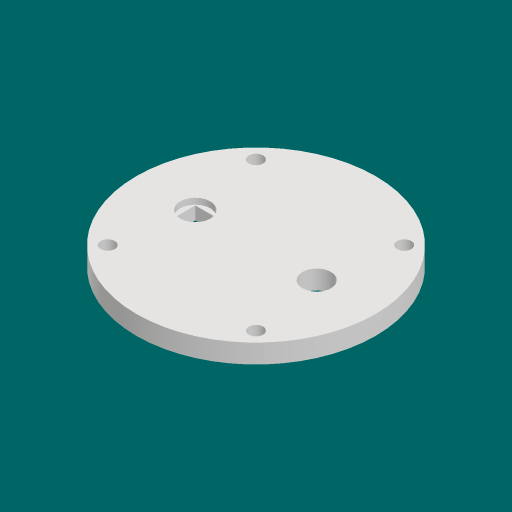
# Autodesk Inventor part: carriage
Saved by Autodesk Inventor 2023.1 (Build 271208000, 208)
## iProperties
Created: 2022-10-10
Part Number: carriage
Material: Generic
Document SubType Name: Modeling
Designer: zac-h
Density: 1 g/cm^3
Appearance: Default
Author: zac-h
Autodesk Inventor part; units mm, degrees
ref_plane "YZ Plane" through (0, 0, 0) normal (1, 0, 0) x (0, 1, 0)
ref_plane "XZ Plane" through (0, 0, 0) normal (0, 1, 0) x (-1, 0, 0)
ref_plane "XY Plane" through (0, 0, 0) normal (0, 0, 1) x (1, 0, 0)
sketch "Sketch1" plane through (0, 0, 0) normal (0, 1, 0) x (-1, 0, 0)
  point P0 (0, 0)
sketch "Sketch2" plane through (0, 0, 0) normal (0, 1, 0) x (-1, 0, 0)
  circle A0 centre (0, 0) radius 4.7625
  circle A1 centre (20.32, 0) radius 40
  line L0 (20.32, -34.925) -> (20.32, 34.925) construction
  line L1 (29.845, -25.4) -> (29.845, 25.4) construction
  line L2 (10.795, 25.4) -> (10.795, -25.4) construction
  arc A2 (10.795, -25.4) -> (29.845, -25.4) centre (20.32, -25.4) ccw construction
  arc A3 (29.845, 25.4) -> (10.795, 25.4) centre (20.32, 25.4) ccw construction
  line L3 (-19.68, 0) -> (60.32, 0) construction
  circle A4 centre (0, 0) radius 20.32 construction
  circle A5 centre (40.64, 0) radius 20.32 construction
  circle A6 centre (20.32, 0) radius 40.64 construction
  line L4 (20.32, 0) -> (48.6043, -28.2843) construction
  line L5 (20.32, 0) -> (60.32, 0) construction
  circle A7 centre (45.1244, -24.8044) radius 2.3812
  circle A8 centre (45.1244, -24.8044) radius 4.9212 construction
  circle A9 centre (45.1244, 24.8044) radius 2.3812
  circle A10 centre (-4.4844, 24.8044) radius 2.3812
  circle A11 centre (-4.4844, -24.8044) radius 2.3812
  line L6 (43.9547, -3.3147) -> (37.3253, -3.3147)
  line L7 (37.3253, -3.3147) -> (37.3253, 3.3147)
  line L8 (37.3253, 3.3147) -> (43.9547, 3.3147)
  line L9 (43.9547, 3.3147) -> (43.9547, -3.3147)
  line L10 (43.9547, -3.3147) -> (37.3253, 3.3147) construction
  line L11 (37.3253, -3.3147) -> (43.9547, 3.3147) construction
  circle A12 centre (40.64, 0) radius 5.0254
  dimension "d5" = 40.64
  dimension "d0" = 9.525
  dimension "d1" = 80
  dimension "d2" = 19.05
  dimension "d3" = 69.85
  dimension "d6" = 81.28
  dimension "d7" = 45
  dimension "d8" = 4.7625
  dimension "d9" = 2.54
  dimension "d12" = 360
  dimension "d16" = 6.6294
  dimension "d18" = 10.0508
  constraints: 26 end point, 10 centre point, 9 point on circle, 5 coincident, 5 point on line, 4 midpoint, 4 tangent, 3 horizontal, 3 horizontal alignment, 3 parallel, 2 equal length, 1 perpendicular, 1 vertical, 17 other
  measures "d0" diameter of A0
  measures "d1" diameter of A1
  measures "d2" diameter of A3
  measures "d3" distance of L0.start L0.end
  measures "d6" diameter of A6
  measures "d7" angle of L4 L5
  measures "d8" diameter of A7
  measures "d16" distance of L7.end L8.end
  measures "d18" diameter of A12
extrude "Extrusion1" add sketch "Sketch2" along normal blind 6.35 contours A1 | A12
sketch "Sketch3" plane through (-20.32, 6.35, 0) normal (0, 1, 0) x (1, 0, 0)
  circle A0 centre (-20.32, 0) radius 5.0254
  point P0 (20.32, 0)
  dimension "d19" = 10.0508
  constraints: 1 centre point
  measures "d19" diameter of A0
extrude "Extrusion2" cut sketch "Sketch3" against normal blind 2
body "Solid1"
